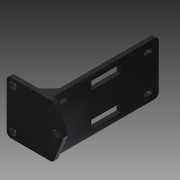
# Autodesk Inventor part: Sonar Mount
Saved by Autodesk Inventor 2015 (Build 190159000, 159)
## iProperties
Created: 2016-02-20
Part Number: Sonar Mount
Material: ABS Plastic
Document SubType Name: Modeling
Designer: 23902
Density: 1.06 g/cm^3
Appearance: Smooth - White
Mass: 2.17586 g
Surface Area: 27.3546 cm^2
Volume: 2.0527 cm^3
Author: 23902
Autodesk Inventor part; units mm, degrees
ref_plane "YZ Plane" through (0, 0, 0) normal (1, 0, 0) x (0, 1, 0)
ref_plane "XZ Plane" through (0, 0, 0) normal (0, 1, 0) x (-1, 0, 0)
ref_plane "XY Plane" through (0, 0, 0) normal (0, 0, 1) x (1, 0, 0)
sketch "Sketch1" plane through (0, 0, 0) normal (0, 1, 0) x (-1, 0, 0)
  line L0 (-10, -12.5) -> (-10, 12.5)
  line L1 (-10, 12.5) -> (10, 12.5)
  line L2 (10, 12.5) -> (10, -12.5)
  line L3 (10, -12.5) -> (-10, -12.5)
  line L4 (-10, -12.5) -> (10, 12.5) construction
  line L5 (-10, 12.5) -> (10, -12.5) construction
  line L6 (-10, -12.5) -> (-10.6459, -12.5)
  line L7 (-10, 12.5) -> (-10.6459, 12.5)
  line L8 (-16.7029, -0.7428) -> (-12.5029, -11.2428)
  line L9 (-12.5029, 11.2428) -> (-16.7029, 0.7428)
  circle A0 centre (-13.5, 0) radius 1.6
  arc A1 (-16.7029, 0.7428) -> (-16.7029, -0.7428) centre (-14.8459, 0) ccw
  arc A2 (-10.6459, 12.5) -> (-12.5029, 11.2428) centre (-10.6459, 10.5) ccw
  arc A3 (-12.5029, -11.2428) -> (-10.6459, -12.5) centre (-10.6459, -10.5) ccw
  point P0 (0, 0)
  point P1 (-12, -12.5)
  point P2 (-12, 12.5)
  dimension "d1" = 20
  dimension "d63" = 2
  dimension "d64" = 2
  dimension "d66" = 3.2
  dimension "d67" = 2
  constraints: 20 end point, 6 point on circle, 6 tangent, 4 centre point, 4 point on line, 2 equal radius, 2 horizontal, 2 midpoint, 2 parallel, 1 perpendicular, 1 vertical
  measures "d1" distance of L0.end L1.end
  measures "d63" distance of L0.start point (-12, -12.5)
  measures "d64" distance of L0.end point (-12, 12.5)
  measures "d66" diameter of A0
  measures "d67" radius of A1
extrude "Extrusion1" add sketch "Sketch1" along normal blind 2
sketch "Sketch2" plane through (0, 2, 0) normal (0, 1, 0) x (1, 0, 0)
  line L0 (10, 12.5) -> (10, -12.5)
  line L1 (10, -12.5) -> (8, -12.5)
  line L2 (8, -12.5) -> (8, 12.5)
  line L3 (8, 12.5) -> (10, 12.5)
  line L4 (10, -12.5) -> (10, 12.5)
  point P0 (0, 0)
  dimension "d4" = 2
  constraints: 10 end point
  measures "d4" distance of L0.end L1.end
extrude "Extrusion2" add sketch "Sketch2" along normal blind 50
sketch "Sketch3" plane through (8, 2, -12.5) normal (-1, 0, 0) x (0, 0, 1)
  line L0 (0, 0) -> (25, 0) projected
  line L1 (2.5, 2.5) -> (2.5, 47.5)
  line L2 (2.5, 47.5) -> (22.5, 47.5)
  line L3 (22.5, 47.5) -> (22.5, 2.5)
  line L4 (22.5, 2.5) -> (2.5, 2.5)
  line L5 (2.5, 2.5) -> (4, 2.5)
  line L6 (22.5, 2.5) -> (21, 2.5)
  line L7 (22.5, 25) -> (22.5, 32)
  line L8 (22.5, 32) -> (18.5, 32)
  line L9 (18.5, 32) -> (18.5, 18)
  line L10 (18.5, 18) -> (22.5, 18)
  line L11 (2.5, 25) -> (2.5, 32)
  line L12 (2.5, 32) -> (6.5, 32)
  line L13 (6.5, 32) -> (6.5, 18)
  line L14 (6.5, 18) -> (2.5, 18)
  line L15 (3, 46) -> (3, 44)
  line L16 (5, 46) -> (5, 44)
  arc A0 (5, 46) -> (3, 46) centre (4, 46) ccw
  arc A1 (3, 44) -> (5, 44) centre (4, 44) ccw
  line L17 (20, 46) -> (20, 44)
  line L18 (22, 46) -> (22, 44)
  arc A2 (22, 46) -> (20, 46) centre (21, 46) ccw
  arc A3 (20, 44) -> (22, 44) centre (21, 44) ccw
  line L19 (3, 6) -> (3, 4)
  line L20 (5, 6) -> (5, 4)
  arc A4 (5, 6) -> (3, 6) centre (4, 6) ccw
  arc A5 (3, 4) -> (5, 4) centre (4, 4) ccw
  line L21 (20, 6) -> (20, 4)
  line L22 (22, 6) -> (22, 4)
  arc A6 (22, 6) -> (20, 6) centre (21, 6) ccw
  arc A7 (20, 4) -> (22, 4) centre (21, 4) ccw
  point P0 (12.5, -2)
  point P1 (2.5, 43)
  point P2 (22.5, 43)
  point P3 (2.5, 7)
  point P4 (22.5, 7)
  dimension "d10" = 45
  dimension "d11" = 20
  dimension "d42" = 4
  dimension "d43" = 14
  dimension "d44" = 2
  dimension "d45" = 2
  dimension "d46" = 2
  dimension "d47" = 2
  dimension "d48" = 2
  dimension "d49" = 2
  dimension "d50" = 2
  dimension "d51" = 2
  constraints: 44 end point, 16 point on circle, 12 tangent, 10 point on line, 9 vertical, 8 centre point, 6 perpendicular, 2 midpoint, 2 parallel
  measures "d10" distance of L1.start L1.end
  measures "d11" distance of L1.end L2.end
  measures "d42" distance of L11.end L12.end
  measures "d43" distance of L12.end L13.end
  measures "d44" distance of L15.start L15.end
  measures "d45" distance of L16.start L16.end
  measures "d46" distance of L17.start L17.end
  measures "d47" distance of L18.start L18.end
  measures "d48" distance of L19.start L19.end
  measures "d49" distance of L20.start L20.end
  measures "d50" distance of L21.start L21.end
  measures "d51" distance of L22.start L22.end
extrude "Extrusion3" cut sketch "Sketch3" against normal blind 2 contours L1 L12 L13 L14 | L10 L9 L8 L3 | A0 L16 A1 L15 | A2 L18 A3 L17 | A4 L20 A5 L19 | A6 L22 A7 L21
sketch "Sketch5" plane through (0, 2, 0) normal (0, 1, 0) x (1, 0, 0)
  line L0 (10.6459, 12.5) -> (-10, 12.5) projected
  line L1 (8, 12.5) -> (3, 12.5)
  line L2 (3, 12.5) -> (3, 10.5)
  line L3 (3, 10.5) -> (8, 10.5)
  line L4 (8, 10.5) -> (8, 12.5)
  line L5 (-10, -12.5) -> (8, -12.5) projected
  line L6 (8, -12.5) -> (3, -12.5)
  line L7 (3, -12.5) -> (3, -10.5)
  line L8 (3, -10.5) -> (8, -10.5)
  line L9 (8, -10.5) -> (8, -12.5)
  point P0 (0, 0)
  point P1 (10, 12.5)
  point P2 (10.9055, 12.5)
  dimension "d22" = 5
  dimension "d23" = 2
  dimension "d24" = 5
  dimension "d25" = 2
  constraints: 16 end point, 4 parallel, 2 perpendicular, 2 point on line
  measures "d22" distance of L1.start L1.end
  measures "d23" distance of L2.end L1.end
  measures "d24" distance of L5.end L6.end
  measures "d25" distance of L6.end L7.end
extrude "Extrusion4" add sketch "Sketch5" along normal blind 5
chamfer "Chamfer1" distance 5 angle 45 2 edges at (3, 7, -11.5) (3, 7, 11.5)
sketch "Sketch6" plane through (0, 2, 0) normal (0, 1, 0) x (1, 0, 0)
  line L0 (-10, -12.5) -> (-7, -12.5)
  line L1 (-10, -12.5) -> (3, -12.5) projected
  line L2 (-7, -12.5) -> (-7, -9.5)
  circle A0 centre (-7, -9.5) radius 1.6
  line L3 (-10, 12.5) -> (-7, 12.5)
  line L4 (3, 12.5) -> (-10, 12.5) projected
  line L5 (-7, 12.5) -> (-7, 9.5)
  circle A1 centre (-7, 9.5) radius 1.6
  point P0 (0, 0)
  dimension "d31" = 3
  dimension "d32" = 3
  dimension "d33" = 3.2
  dimension "d34" = 3
  dimension "d35" = 3
  dimension "d36" = 3.2
  constraints: 8 end point, 2 centre point, 2 coincident, 2 point on line, 1 perpendicular, 1 vertical
  measures "d31" distance of L0.start L0.end
  measures "d32" distance of L0.end L2.end
  measures "d33" diameter of A0
  measures "d34" distance of L3.start L3.end
  measures "d35" distance of L3.end L5.end
  measures "d36" diameter of A1
extrude "Extrusion5" cut sketch "Sketch6" against normal blind 5
fillet "Fillet1" radius 2 4 edges at (-10, 1, 12.5) (-10, 1, -12.5) (9, 52, 12.5) (9, 52, -12.5)
equation "\"d20\" = d49"
body "Solid1"
